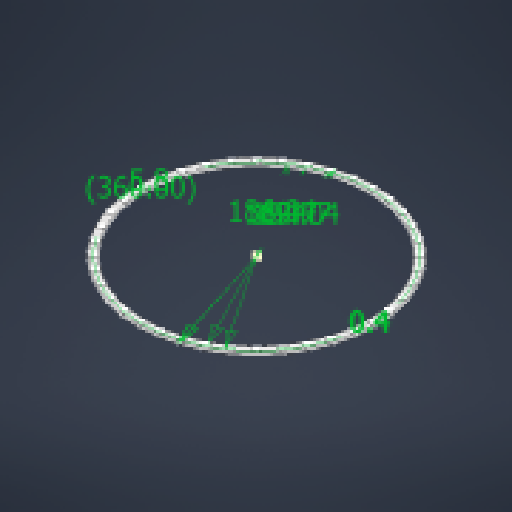
# Autodesk Inventor part: thrust_bearing_v1
Saved by Autodesk Inventor 2026.1 (Build 301233020, 233B)
## iProperties
Created: 2025-12-01
Part Number: thrust_bearing_v1
Material: 일반
Document SubType Name: Modeling
Designer: jaewook
Density: 1 g/cm^3
Appearance: 기본값
Author: jaewook
Autodesk Inventor part; units mm, degrees
ref_plane "YZ Plane" through (0, 0, 0) normal (1, 0, 0) x (0, 1, 0)
ref_plane "XZ Plane" through (0, 0, 0) normal (0, 1, 0) x (-1, 0, 0)
ref_plane "XY Plane" through (0, 0, 0) normal (0, 0, 1) x (1, 0, 0)
sketch "스케치1" plane through (0, 0, 0) normal (0, 1, 0) x (-1, 0, 0)
  circle A0 centre (0, 0) radius 91.35
  circle A1 centre (0, 0) radius 97.02 construction
  circle A2 centre (0, 0) radius 97.35
  circle A3 centre (0, 0) radius 93.02 construction
  line L0 (91.35, 0) -> (97.35, 0) construction
  circle A4 centre (94.35, 0) radius 2.9
  circle A5 centre (93.188395, 14.759592) radius 2.9
  circle A6 centre (89.732182, 29.155753) radius 2.9
  circle A7 centre (84.066466, 42.834004) radius 2.9
  circle A8 centre (76.330753, 55.457539) radius 2.9
  circle A9 centre (66.715525, 66.715525) radius 2.9
  circle A10 centre (55.457539, 76.330753) radius 2.9
  circle A11 centre (42.834004, 84.066466) radius 2.9
  circle A12 centre (29.155753, 89.732182) radius 2.9
  circle A13 centre (14.759592, 93.188395) radius 2.9
  circle A14 centre (0, 94.35) radius 2.9
  circle A15 centre (-14.759592, 93.188395) radius 2.9
  circle A16 centre (-29.155753, 89.732182) radius 2.9
  circle A17 centre (-42.834004, 84.066466) radius 2.9
  circle A18 centre (-55.457539, 76.330753) radius 2.9
  circle A19 centre (-66.715525, 66.715525) radius 2.9
  circle A20 centre (-76.330753, 55.457539) radius 2.9
  circle A21 centre (-84.066466, 42.834004) radius 2.9
  circle A22 centre (-89.732182, 29.155753) radius 2.9
  circle A23 centre (-93.188395, 14.759592) radius 2.9
  circle A24 centre (-94.35, 0) radius 2.9
  circle A25 centre (-93.188395, -14.759592) radius 2.9
  circle A26 centre (-89.732182, -29.155753) radius 2.9
  circle A27 centre (-84.066466, -42.834004) radius 2.9
  circle A28 centre (-76.330753, -55.457539) radius 2.9
  circle A29 centre (-66.715525, -66.715525) radius 2.9
  circle A30 centre (-55.457539, -76.330753) radius 2.9
  circle A31 centre (-42.834004, -84.066466) radius 2.9
  circle A32 centre (-29.155753, -89.732182) radius 2.9
  circle A33 centre (-14.759592, -93.188395) radius 2.9
  circle A34 centre (0, -94.35) radius 2.9
  circle A35 centre (14.759592, -93.188395) radius 2.9
  circle A36 centre (29.155753, -89.732182) radius 2.9
  circle A37 centre (42.834004, -84.066466) radius 2.9
  circle A38 centre (55.457539, -76.330753) radius 2.9
  circle A39 centre (66.715525, -66.715525) radius 2.9
  circle A40 centre (76.330753, -55.457539) radius 2.9
  circle A41 centre (84.066466, -42.834004) radius 2.9
  circle A42 centre (89.732182, -29.155753) radius 2.9
  circle A43 centre (93.188395, -14.759592) radius 2.9
  circle A44 centre (0, 0) radius 91.75
  circle A45 centre (0, 0) radius 92.62
  dimension "d0" = 182.7
  dimension "d2" = 194.7
  dimension "d1" = 194.04
  dimension "d3" = 186.04
  dimension "d4" = 5.8
  dimension "d7" = 360
  dimension "d16" = 0.4
  dimension "d17" = 0.4
  constraints: 44 centre point, 4 coincident, 3 horizontal alignment, 2 end point, 1 horizontal, 1 midpoint, 85 other
  measures "d1" diameter of A1
  measures "d3" diameter of A3
  measures "d4" diameter of A4
  measures "d17" radial gap between concentric circles of A3 A45
sketch "스케치1 outline for 돌출1" plane through (0, 0, 0) normal (0, 1, 0) x (-1, 0, 0)
  circle A0 centre (0, 0) radius 97.35
  circle A1 centre (-55.457539, -76.330753) radius 2.9
  circle A2 centre (-76.330753, -55.457539) radius 2.9
  circle A3 centre (-66.715525, -66.715525) radius 2.9
  circle A4 centre (-29.155753, -89.732182) radius 2.9
  circle A5 centre (-42.834004, -84.066466) radius 2.9
  circle A6 centre (-14.759592, -93.188395) radius 2.9
  circle A7 centre (0, -94.35) radius 2.9
  circle A8 centre (-84.066466, -42.834004) radius 2.9
  circle A9 centre (-89.732182, -29.155753) radius 2.9
  circle A10 centre (-93.188395, -14.759592) radius 2.9
  circle A11 centre (0, 0) radius 91.35
  circle A12 centre (14.759592, -93.188395) radius 2.9
  circle A13 centre (29.155753, -89.732182) radius 2.9
  circle A14 centre (42.834004, -84.066466) radius 2.9
  circle A15 centre (55.457539, -76.330753) radius 2.9
  circle A16 centre (66.715525, -66.715525) radius 2.9
  circle A17 centre (76.330753, -55.457539) radius 2.9
  circle A18 centre (84.066466, -42.834004) radius 2.9
  circle A19 centre (89.732182, -29.155753) radius 2.9
  circle A20 centre (93.188395, -14.759592) radius 2.9
  circle A21 centre (94.35, 0) radius 2.9
  circle A22 centre (-94.35, 0) radius 2.9
  circle A23 centre (-93.188395, 14.759592) radius 2.9
  circle A24 centre (-89.732182, 29.155753) radius 2.9
  circle A25 centre (-84.066466, 42.834004) radius 2.9
  circle A26 centre (-76.330753, 55.457539) radius 2.9
  circle A27 centre (-66.715525, 66.715525) radius 2.9
  circle A28 centre (-55.457539, 76.330753) radius 2.9
  circle A29 centre (-42.834004, 84.066466) radius 2.9
  circle A30 centre (-29.155753, 89.732182) radius 2.9
  circle A31 centre (-14.759592, 93.188395) radius 2.9
  circle A32 centre (0, 94.35) radius 2.9
  circle A33 centre (93.188395, 14.759592) radius 2.9
  circle A34 centre (89.732182, 29.155753) radius 2.9
  circle A35 centre (84.066466, 42.834004) radius 2.9
  circle A36 centre (14.759592, 93.188395) radius 2.9
  circle A37 centre (42.834004, 84.066466) radius 2.9
  circle A38 centre (29.155753, 89.732182) radius 2.9
  circle A39 centre (66.715525, 66.715525) radius 2.9
  circle A40 centre (76.330753, 55.457539) radius 2.9
  circle A41 centre (55.457539, 76.330753) radius 2.9
extrude "돌출1" add sketch "스케치1 outline for 돌출1" along normal mid plane 2
sketch "스케치2" plane through (0, 0, 0) normal (1, 0, 0) x (0, 1, 0)
  line L0 (1, 97.25) -> (1, 91.45) projected
  line L1 (-1, 91.45) -> (-1, 97.25) projected
  line L2 (1, 97.25) -> (-1, 97.25) projected
  line L3 (1, 91.45) -> (-1, 91.45) projected
  line L4 (0, 97.25) -> (0, 91.45)
  circle A0 centre (0, 94.35) radius 2.8
  point P0 (0, 0)
  point P1 (0, 97.15)
  point P2 (0, 91.55)
  dimension "d11" = 5.6
  constraints: 3 midpoint, 2 end point, 1 centre point
  measures "d11" diameter of A0
